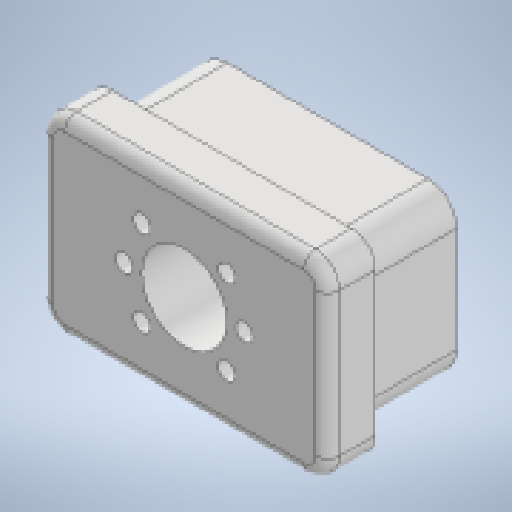
# Autodesk Inventor part: 2x3_Spacer
Saved by Autodesk Inventor 2023 (Build 270158000, 158)
## iProperties
Created: 2022-05-03
Part Number: 2x3_Spacer
Material: Generic
Document SubType Name: Modeling
Designer: plebbb
Density: 1 g/cm^3
Appearance: Default
Author: plebbb
Autodesk Inventor part; units mm, degrees
ref_plane "YZ Plane" through (0, 0, 0) normal (1, 0, 0) x (0, 1, 0)
ref_plane "XZ Plane" through (0, 0, 0) normal (0, 1, 0) x (-1, 0, 0)
ref_plane "XY Plane" through (0, 0, 0) normal (0, 0, 1) x (1, 0, 0)
sketch "Sketch1" plane through (0, 0, 0) normal (0, 0, 1) x (1, 0, 0)
  line L0 (7.62, 0) -> (60.96, 0)
  line L1 (68.58, 7.62) -> (68.58, 35.56)
  line L2 (60.96, 43.18) -> (7.62, 43.18)
  line L3 (0, 35.56) -> (0, 7.62)
  arc A0 (7.62, 43.18) -> (0, 35.56) centre (7.62, 35.56) ccw
  arc A1 (0, 7.62) -> (7.62, 0) centre (7.62, 7.62) ccw
  arc A2 (68.58, 35.56) -> (60.96, 43.18) centre (60.96, 35.56) ccw
  arc A3 (60.96, 0) -> (68.58, 7.62) centre (60.96, 7.62) ccw
  point P0 (0, 0)
  point P1 (68.58, 43.18)
  point P2 (68.58, 0)
  point P3 (0, 43.18)
  dimension "d0" = 68.58
  dimension "d1" = 43.18
  dimension "d3" = 7.62
  constraints: 8 end point, 8 point on circle, 8 point on line, 8 tangent, 4 centre point, 3 equal radius, 2 parallel, 1 horizontal, 1 perpendicular
  measures "d0" distance of point (68.58, 43.18) point (0, 43.18)
  measures "d1" distance of point (68.58, 0) point (68.58, 43.18)
  measures "d3" radius of A0
extrude "Extrusion1" add sketch "Sketch1" along normal blind 25.4
sketch "Sketch2" plane through (0, 0, 25.4) normal (0, 0, 1) x (1, 0, 0)
  line L0 (2.54, -3.81) -> (66.04, -3.81)
  line L1 (72.39, 2.54) -> (72.39, 40.64)
  line L2 (66.04, 46.99) -> (2.54, 46.99)
  line L3 (-3.81, 40.64) -> (-3.81, 2.54)
  line L4 (60.96, 43.18) -> (7.62, 43.18) construction
  line L5 (0, 35.56) -> (0, 7.62) construction
  line L6 (7.62, 0) -> (60.96, 0) construction
  line L7 (68.58, 7.62) -> (68.58, 35.56) construction
  arc A0 (2.54, 46.99) -> (-3.81, 40.64) centre (2.54, 40.64) ccw
  arc A1 (-3.81, 2.54) -> (2.54, -3.81) centre (2.54, 2.54) ccw
  arc A2 (66.04, -3.81) -> (72.39, 2.54) centre (66.04, 2.54) ccw
  arc A3 (72.39, 40.64) -> (66.04, 46.99) centre (66.04, 40.64) ccw
  point P0 (0, 0)
  point P1 (72.39, 46.99)
  point P2 (72.39, -3.81)
  point P3 (-3.81, 46.99)
  point P4 (34.29, 46.99)
  point P5 (34.29, 43.18)
  point P6 (68.58, 21.59)
  point P7 (72.39, 21.59)
  dimension "d6" = 76.2
  dimension "d7" = 50.8
  dimension "d8" = 6.35
  constraints: 8 end point, 8 point on circle, 8 tangent, 6 point on line, 4 centre point, 4 midpoint, 3 equal radius, 2 parallel, 1 horizontal, 1 horizontal alignment, 1 perpendicular, 1 vertical alignment
  measures "d6" distance of point (72.39, 46.99) point (-3.81, 46.99)
  measures "d7" distance of point (72.39, -3.81) point (72.39, 46.99)
  measures "d8" radius of A0
extrude "Extrusion2" add sketch "Sketch2" along normal blind 12.7
fillet "Fillet1" radius 3.175 8 edges at (-1.9501, 45.1301, 38.1) (-3.81, 21.59, 38.1) (-1.9501, -1.9501, 38.1) (34.29, -3.81, 38.1) (70.5301, -1.9501, 38.1) (72.39, 21.59, 38.1) (70.5301, 45.1301, 38.1) (34.29, 46.99, 38.1)
sketch "Sketch3" plane through (0, 0, 38.1) normal (0, 0, 1) x (1, 0, 0)
  circle A0 centre (34.29, 21.59) radius 11.25
  line L0 (-0.635, 2.54) -> (-0.635, 40.64) construction
  line L1 (2.54, 43.815) -> (66.04, 43.815) construction
  circle A1 centre (34.29, 21.59) radius 16 construction
  circle A2 centre (45.6037, 32.9037) radius 2.3
  circle A3 centre (18.29, 21.59) radius 2.3
  circle A4 centre (45.6037, 10.2763) radius 2.3
  circle A5 centre (50.29, 21.59) radius 2.3
  circle A6 centre (22.9763, 32.9037) radius 2.3
  circle A7 centre (22.9763, 10.2763) radius 2.3
  line L2 (22.9763, 32.9037) -> (34.29, 21.59) construction
  line L3 (34.29, 21.59) -> (18.29, 21.59) construction
  point P0 (0, 0)
  point P1 (34.29, 43.815)
  point P2 (-0.635, 21.59)
  dimension "d12" = 22.5
  dimension "d13" = 32
  dimension "d14" = 4.6
  dimension "d15" = 45
  constraints: 8 centre point, 6 point on circle, 5 equal radius, 4 end point, 4 horizontal alignment, 3 vertical alignment, 2 midpoint, 1 coincident, 1 horizontal
  measures "d12" diameter of A0
  measures "d13" diameter of A1
  measures "d14" diameter of A3
  measures "d15" angle of L3 L2
extrude "Extrusion3" cut sketch "Sketch3" against normal up to surface (38.1 mm away)
body "Solid1"
